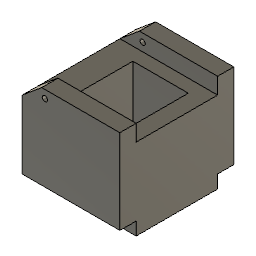
FingerJoints (Autodesk Fusion 360 design; units mm, degrees)
part number: 2025-11-11-21-26-34-936
Autodesk Fusion 360 part; units mm, degrees
sketch "Sketch1" plane through (0, 0, 0) normal (0, 0, 1) x (1, 0, 0)
  line L0 (0, 0) -> (30, 0)
  line L1 (30, 0) -> (30, 35)
  line L2 (30, 35) -> (0, 35)
  line L3 (0, 35) -> (0, 0)
  dimension "d1" = 30
  dimension "d2" = 35
  constraint horizontal L0
  constraint vertical L1
  constraint horizontal L2
  constraint vertical L3
  constraint coincident L0.start L3.end
  measures "d1" distance of L0.start L0.end
  measures "d2" distance of L0.start L2.end
extrude "Extrude1" add sketch "Sketch1" along normal blind 30
sketch "Sketch2" plane through (0, 0, 0) normal (0, 0, -1) x (1, 0, 0)
  line L0 (0, 0) -> (0, -35)
  line L1 (0, -35) -> (30, -35)
  line L2 (30, -35) -> (30, 0)
  line L3 (30, 0) -> (0, 0)
  line L4 (30, 0) -> (0, 0)
  line L5 (0, 0) -> (0, -5)
  line L6 (0, -5) -> (30, -5)
  line L7 (30, -5) -> (30, 0)
  line L8 (30, -35) -> (0, -35)
  line L9 (0, -35) -> (0, -30)
  line L10 (0, -30) -> (30, -30)
  line L11 (30, -30) -> (30, -35)
  constraint horizontal L4
  constraint vertical L5
  constraint horizontal L6
  constraint vertical L7
  constraint coincident L0 L5.end
  constraint coincident L2.end L3.start
  constraint horizontal L8
  constraint vertical L9
  constraint horizontal L10
  constraint vertical L11
  constraint coincident L0 L9.end
  constraint coincident L1.end L2.start
extrude "Extrude2" cut sketch "Sketch2" against normal blind 4 contours L0 L2 L3 L4 L5 L6 L7 | L0 L1 L2 L8 L9 L10 L11
sketch "Sketch3" plane through (0, 5, 0) normal (0, -1, 0) x (1, 0, 0)
  line L0 (0, 0) -> (30, 0)
  line L1 (30, 0) -> (30, 4)
  line L2 (30, 4) -> (0, 4)
  line L3 (0, 4) -> (0, 0)
  line L4 (0, 4) -> (5, 0)
  constraint coincident L2.end L3.start
  constraint coincident L0 L4.end
extrude "Extrude3" cut sketch "Sketch3" against normal blind 100 contours L0 L3 L4
sketch "Sketch4" plane through (0, 5, 0) normal (0, -1, 0) x (1, 0, 0)
  line L0 (0, 4) -> (5, 0)
  line L1 (5, 0) -> (30, 0)
  line L2 (30, 0) -> (30, 4)
  line L3 (30, 4) -> (0, 4)
  circle A0 centre (7, 2.5) radius 1
  dimension "d9" = 2
  measures "d9" diameter of A0
sketch "Sketch5" plane through (0, 0, 0) normal (0, 0, -1) x (1, 0, 0)
  line L0 (5, -5) -> (5, -30)
  line L1 (5, -30) -> (30, -30)
  line L2 (30, -30) -> (30, -5)
  line L3 (30, -5) -> (5, -5)
  line L4 (25, -26) -> (10, -26)
  line L5 (10, -26) -> (10, -9)
  line L6 (10, -9) -> (25, -9)
  line L7 (25, -9) -> (25, -26)
  constraint horizontal L4
  constraint vertical L5
  constraint horizontal L6
  constraint vertical L7
extrude "Extrude5" cut sketch "Sketch5" against normal blind 100 contours L4 L5 L6 L7
sketch "Sketch6" plane through (25, 0, 0) normal (-1, 0, 0) x (0, -1, 0)
  line L0 (-9, 30) -> (-26, 30)
  line L1 (-26, 30) -> (-26, 0)
  line L2 (-26, 0) -> (-9, 0)
  line L3 (-9, 0) -> (-9, 30)
  line L4 (-9, 0) -> (-26, 0)
  line L5 (-26, 0) -> (-26, 3)
  line L6 (-26, 3) -> (-9, 3)
  line L7 (-9, 3) -> (-9, 0)
  dimension "d14" = 17
  dimension "d15" = 3
  constraint horizontal L4
  constraint vertical L5
  constraint horizontal L6
  constraint vertical L7
  constraint coincident L2.end L3.start
  measures "d14" distance of L2.end L1.end
  measures "d15" distance of L2.end L6.end
extrude "Extrude6" add sketch "Sketch6" along normal blind 5 contours L1 L2 L3 L4 L5 L6 L7
sketch "Sketch7" plane through (0, 0, 0) normal (0, -1, 0) x (1, 0, 0)
  line L0 (0, 4) -> (30, 4)
  line L1 (30, 4) -> (30, 30)
  line L2 (30, 30) -> (0, 30)
  line L3 (0, 30) -> (0, 4)
  line L4 (0, 25) -> (6, 30)
  constraint coincident L3 L4.start
  constraint coincident L2 L4.end
extrude "Extrude7" cut sketch "Sketch7" against normal blind 100 contours L2 L3 L4
sketch "Sketch8" plane through (0, 0, 30) normal (0, 0, 1) x (-1, 0, 0)
  line L0 (-6, -35) -> (-6, 0)
  line L1 (-6, 0) -> (-30, 0)
  line L2 (-30, 0) -> (-30, -35)
  line L3 (-30, -35) -> (-6, -35)
  line L4 (-10, -9) -> (-10, -26)
  line L5 (-10, -26) -> (-25, -26)
  line L6 (-25, -26) -> (-25, -9)
  line L7 (-25, -9) -> (-10, -9)
  line L8 (-30, -30) -> (0, -30)
  line L9 (0, -30) -> (0, -5)
  line L10 (0, -5) -> (-30, -5)
  line L11 (-30, -5) -> (-30, -30)
  constraint horizontal L8
  constraint vertical L9
  constraint horizontal L10
  constraint vertical L11
  constraint coincident L2 L8.start
extrude "Extrude8" cut sketch "Sketch8" against normal blind 5 contours L0 L2 L8 L10 L11 | L0 L8 L9 L10
sketch "Sketch9" plane through (0, 5, 0) normal (0, -1, 0) x (1, 0, 0)
  line L0 (0, 4) -> (5, 0)
  line L1 (5, 0) -> (30, 0)
  line L2 (30, 0) -> (30, 4)
  line L3 (30, 4) -> (0, 4)
  circle A0 centre (7, 2) radius 0.8
  dimension "d22" = 1.6
  measures "d22" diameter of A0
extrude "Extrude9" cut sketch "Sketch9" against normal blind 100 contours A0
sketch "Sketch10" plane through (0, 0, 0) normal (0, -1, 0) x (1, 0, 0)
  line L0 (6, 30) -> (0, 25)
  line L1 (0, 25) -> (0, 4)
  line L2 (0, 4) -> (30, 4)
  line L3 (30, 4) -> (30, 30)
  line L4 (30, 30) -> (6, 30)
  circle A0 centre (7, 28.5) radius 0.8
  dimension "d25" = 1.6
  measures "d25" diameter of A0
sketch "Sketch11" plane through (0, 0, 0) normal (0, -1, 0) x (1, 0, 0)
  line L0 (6, 30) -> (0, 25)
  line L1 (0, 25) -> (0, 4)
  line L2 (0, 4) -> (30, 4)
  line L3 (30, 4) -> (30, 30)
  line L4 (30, 30) -> (6, 30)
  circle A0 centre (7, 27.545) radius 0.8
  line L5 (7, 27.545) -> (7, 1)
  dimension "d28" = 1.6
  dimension "d29" = 7
  dimension "d30" = 2.455
  constraint coincident A0.centre L5.start
  constraint vertical L5
  measures "d28" diameter of A0
  measures "d29" distance of L1 A0.centre
  measures "d30" distance of L4 A0.centre
extrude "Extrude11" cut sketch "Sketch11" against normal blind 100 contours A0
sketch "Sketch12" plane through (10, 0, 0) normal (1, 0, 0) x (0, 1, 0)
  line L0 (26, 25) -> (9, 25)
  line L1 (9, 25) -> (9, 0)
  line L2 (9, 0) -> (26, 0)
  line L3 (26, 0) -> (26, 25)
  line L4 (26, 0) -> (9, 0)
  line L5 (9, 0) -> (9, 3)
  line L6 (9, 3) -> (26, 3)
  line L7 (26, 3) -> (26, 0)
  dimension "d33" = 17
  dimension "d34" = 3
  constraint horizontal L4
  constraint vertical L5
  constraint horizontal L6
  constraint vertical L7
  constraint coincident L2.end L3.start
  measures "d33" distance of L2.end L1.end
  measures "d34" distance of L2.end L6.end
extrude "Extrude12" add sketch "Sketch12" along normal blind 2 contours L1 L2 L3 L4 L5 L6 L7
extrude "Extrude13" cut 1 faces at (20, 20.3333, 1) along direction (1, 0, 0) blind 2.5
extrude "Extrude14" cut 1 faces at (24.1667, 20.3333, 3) along direction (0, 0, -1) blind 1
extrude "Extrude15" cut 1 faces at (10.6667, 14.6667, 3) along direction (0, 0, -1) blind 1
extrude "Extrude16" cut 2 faces at (10.6667, 14.6667, 2) (24.1667, 20.3333, 2) along direction (0, 0, -1) blind 0.5
extrude "Extrude17" add 1 faces at (12, 14.6667, 0.5) along direction (1, 0, 0) blind 0.5
extrude "Extrude18" cut 1 faces at (10, 20.3333, 9.8333) along direction (-1, 0, 0) blind 2
